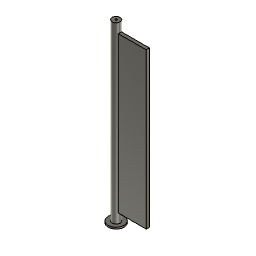
_Grip arm.5dc257c2-be48-415f-a2dd-390b55c8ae94 (Autodesk Fusion 360 design; units mm, degrees)
Autodesk Fusion 360 part; units mm, degrees
sketch "Sketch1" plane through (0, 0, 0) normal (0, 0, 1) x (1, 0, 0)
  circle A0 centre (0, 0) radius 25
  dimension "d1" = 50
  constraint coincident A0.centre origin
  measures "d1" diameter of A0
extrude "Extrude1" add sketch "Sketch1" along normal blind 5
sketch "Sketch2" plane through (0, 0, 5) normal (0, 0, 1) x (-1, 0, 0)
  circle A0 centre (0, 0) radius 25
  circle A1 centre (0, 0) radius 12.5
  dimension "d4" = 25
  constraint concentric A0 A1
  measures "d4" diameter of A1
extrude "Extrude2" add sketch "Sketch2" along normal blind 550 contours A1
sketch "Sketch3" plane through (0, 0, 555) normal (0, 0, 1) x (-1, 0, 0)
  circle A0 centre (0, 0) radius 12.5
  line L0 (0, -5) -> (-100, -5)
  line L1 (-100, -5) -> (-100, 5)
  line L2 (-100, 5) -> (0, 5)
  line L3 (0, 5) -> (0, -5)
  dimension "d7" = 100
  dimension "d8" = 10
  constraint horizontal L0
  constraint vertical L1
  constraint horizontal L2
  constraint vertical L3
  measures "d7" distance of L0.start L0.end
  measures "d8" distance of L0.start L2.end
extrude "Extrude3" add sketch "Sketch3" against normal blind 525 contours A0 L0 L1 L2
extrude "Extrude4" cut sketch "Sketch3" against normal blind 25 contours A0 L0 L1 L2
sketch "Sketch4" plane through (0, 0, 555) normal (0, 0, 1) x (-1, 0, 0)
  circle A0 centre (0, 0) radius 12.5
  circle A1 centre (0, 0) radius 3
  dimension "d13" = 6
  constraint coincident A0.centre A1.centre
  measures "d13" diameter of A1
extrude "Extrude5" cut sketch "Sketch4" against normal blind 10 contours A1
extrude "Extrude6" cut 1 faces at (70.8333, 0, 530) along direction (0, 0, -1) blind 5
extrude "Extrude7" cut 1 faces at (70.8333, 0, 30) along direction (0, 0, 1) blind 5
